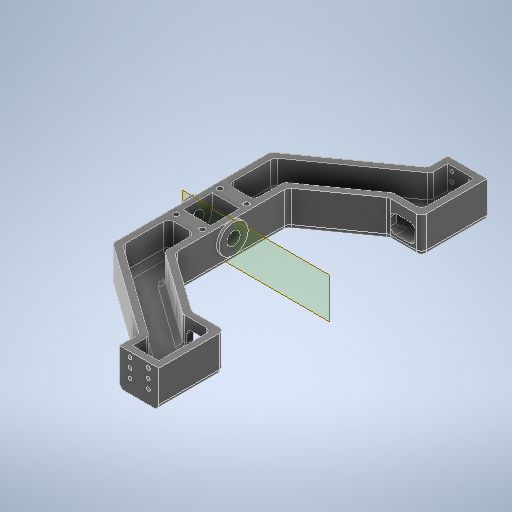
# Autodesk Inventor part: handler_back
Saved by Autodesk Inventor 2025.3 (Build 293356000, 356)
## iProperties
Created: 2026-04-18
Part Number: handler_back
Material: PCTG 20%
Document SubType Name: Modeling
Designer: ksawe
Density: 1.541 g/cm^3
Appearance: Smooth - Black
Author: ksawe
Autodesk Inventor part; units mm, degrees
ref_plane "YZ Plane" through (0, 0, 0) normal (1, 0, 0) x (0, 1, 0)
ref_plane "XZ Plane" through (0, 0, 0) normal (0, 1, 0) x (-1, 0, 0)
sketch "Sketch1" plane through (0, 0, 0) normal (0, 1, 0) x (-1, 0, 0)
  line L0 (-100, 125) -> (-70, 125)
  line L1 (0, 0) -> (-70, 0) construction
  line L2 (-100, 125) -> (-100, 75)
  line L3 (-100, 75) -> (-75, 75)
  line L4 (-70, 125) -> (-70, 110)
  line L5 (-70, 110) -> (0, 60)
  line L6 (0, 60) -> (0, 0)
  line L7 (-75, 75) -> (-30, 42.8571)
  line L8 (-30, 42.8571) -> (-30, 0)
  line L9 (-100, -125) -> (-70, -125)
  line L10 (-100, -125) -> (-100, -75)
  line L11 (-100, -75) -> (-75, -75)
  line L12 (-70, -125) -> (-70, -110)
  line L13 (-70, -110) -> (0, -60)
  line L14 (0, -60) -> (0, 0)
  line L15 (-75, -75) -> (-30, -42.8571)
  line L16 (-30, -42.8571) -> (-30, 0)
  line L17 (-5, 0) -> (-5, 57.4269)
  line L18 (-5, 57.4269) -> (-75, 107.4269)
  line L19 (-75, 107.4269) -> (-75, 120)
  line L20 (-75, 120) -> (-95, 120)
  line L21 (-95, 120) -> (-95, 80)
  line L22 (-95, 80) -> (-73.3977, 80)
  line L23 (-73.3977, 80) -> (-25, 45.4302)
  line L24 (-25, 45.4302) -> (-25, 0)
  line L25 (-25, 0) -> (-25, -45.4302)
  line L26 (-25, -45.4302) -> (-73.3977, -80)
  line L27 (-73.3977, -80) -> (-95, -80)
  line L28 (-95, -80) -> (-95, -120)
  line L29 (-95, -120) -> (-75, -120)
  line L30 (-75, -120) -> (-75, -107.4269)
  line L31 (-75, -107.4269) -> (-5, -57.4269)
  line L32 (-5, -57.4269) -> (-5, 0)
  dimension "d0" = 125
  dimension "d5" = 30
  dimension "d20" = 50
  dimension "d21" = 25
  dimension "d23" = 15
  dimension "d26" = 100
  dimension "d27" = 60
  dimension "d29" = 30
  dimension "d32" = 70
  dimension "d33" = 5
  constraints: 66 end point, 7 symmetric about line, 4 coincident, 4 vertical, 2 horizontal, 2 parallel, 1 horizontal alignment, 15 other
  measures "d0" distance between parallel lines of L1 L0
  measures "d5" distance of L0.start L0.end
  measures "d20" distance of L0.start L2.end
  measures "d21" distance of L2.end L3.end
  measures "d23" distance of L0.end L4.end
  measures "d26" distance between parallel lines of L2 L6
  measures "d27" distance of L5.end L6.end
  measures "d29" distance between parallel lines of L8 L6
  measures "d32" distance of L1.start L1.end
  measures "d33" distance between parallel lines of L6 L17
extrude "Extrusion3" add sketch "Sketch1" against normal blind 6 contours L0 L4 L5 L6 L14 L13 L12 L9 L10 L11 L15 L16 L8 L7 L3 L2 | L32 L31 L30 L29 L28 L27 L26 L25 L24 L23 L22 L21 L20 L19 L18 L17
extrude "Extrusion4" add sketch "Sketch1" along normal blind 22
sketch "Szkic3" plane through (0, 0, 0) normal (0, 1, 0) x (1, 0, 0)
  line L0 (25.5, 11.05) -> (4.5, 11.05)
  line L1 (4.5, 11.05) -> (4.5, -11.05)
  line L2 (4.5, -11.05) -> (25.5, -11.05)
  line L3 (25.5, -11.05) -> (25.5, 11.05)
  line L4 (25.5, 11.05) -> (4.5, -11.05) construction
  line L5 (4.5, 11.05) -> (25.5, -11.05) construction
  line L6 (5, -57.4269) -> (5, 57.4269) projected
  line L7 (5, -22.55) -> (25, -22.55)
  line L8 (25, -45.4302) -> (25, 45.4302) projected
  line L9 (5, 22.55) -> (25, 22.55)
  line L10 (5, 0) -> (25, 0) construction
  point P0 (0, 0)
  point P1 (15, 0)
  point P2 (5, 11.05)
  point P3 (25, 11.05)
  point P4 (25, -11.05)
  point P5 (5, -11.05)
  dimension "d34" = 21
  dimension "d35" = 10
  dimension "d36" = 22.1
  dimension "d37" = 11.5
  constraints: 18 end point, 4 midpoint, 4 point on line, 2 horizontal, 2 parallel, 2 perpendicular, 1 horizontal alignment, 1 other
  measures "d34" distance of L2.end L1.end
  measures "d35" distance from line of L6 point (15, 0)
  measures "d36" distance between parallel lines of L0 L2
  measures "d37" distance between parallel lines of L2 L7
extrude "Wyciągnięcie proste6" add sketch "Szkic3" along normal blind 22 contours L0 L6 L9 L8 | L8 L7 L6 L2
sketch "Szkic4" plane through (30, -6, 42.8571) normal (1, 0, 0) x (0, 0, -1)
  circle A0 centre (42.8571, 16.95) radius 5
  circle A1 centre (42.8571, 16.95) radius 11.05
  line L0 (0, 28) -> (85.7143, 28) projected
  point P0 (42.8571, 6)
  dimension "d40" = 10
  dimension "d41" = 22.1
  constraints: 2 centre point, 2 coincident, 1 tangent, 1 vertical alignment
  measures "d40" diameter of A0
  measures "d41" diameter of A1
extrude "Wyciągnięcie proste7" add sketch "Szkic4" along normal blind 2
extrude "Wyciągnięcie proste8" cut sketch "Szkic4" against normal through all contours A0
ref_plane "Płaszczyzna konstrukcyjna1" through (15, 0, -11.05) normal (1, 0, 0) x (0, 0, -1)
mirror "Odbij1" about plane through (15, 0, -11.05) normal (1, 0, 0) of "Wyciągnięcie proste7"
sketch "Szkic9" plane through (0, 22, 0) normal (0, 1, 0) x (1, 0, 0)
  circle A0 centre (5, -16.8) radius 1.5
  circle A1 centre (5, 16.8) radius 1.5
  circle A2 centre (25, -16.8) radius 1.5
  circle A3 centre (25, 16.8) radius 1.5
  line L0 (25, 11.05) -> (25, -11.05) projected
  line L1 (25, -11.05) -> (5, -11.05) projected
  line L2 (5, -11.05) -> (5, 11.05) projected
  line L3 (5, 11.05) -> (25, 11.05) projected
  line L4 (0, 0) -> (0, -60) projected
  line L5 (5, 0) -> (25, 0)
  line L6 (15, -11.05) -> (15, 11.05)
  dimension "d52" = 3
  dimension "d83" = 5.75
  dimension "d84" = 5
  constraints: 4 centre point, 4 end point, 4 midpoint, 3 other
  measures "d52" diameter of A0
  measures "d83" distance from line of L1 A0.centre
  measures "d84" distance from line of L4 A0.centre
hole "Otwór1" at (5, 22, 16.8) at (25, 22, 16.8) at (25, 22, -16.8) at (5, 22, -16.8) direction (0, -1, 0) diameter 4 depth 7 countersink diameter 4.2 countersink angle 90
sketch "Szkic10" plane through (95, 0, 120) normal (0, 0, -1) x (-1, 0, 0)
  circle A0 centre (3, 18.25) radius 1.5
  line L0 (0, 0) -> (0, 22) projected
  line L1 (0, 22) -> (20, 22) projected
  circle A1 centre (17, 18.25) radius 1.5
  circle A2 centre (3, 11.25) radius 1.5
  circle A3 centre (17, 11.25) radius 1.5
  circle A4 centre (3, 4.25) radius 1.5
  circle A5 centre (17, 4.25) radius 1.5
  line L2 (10, 22) -> (10, 0) construction
  line L3 (20, 0) -> (0, 0) projected
  point P0 (95, 0)
  dimension "d60" = 3
  dimension "d64" = 14
  dimension "d67" = 7
  dimension "d70" = 3.75
  constraints: 6 centre point, 2 end point, 2 midpoint, 1 horizontal, 1 vertical, 11 other
  measures "d60" diameter of A0
  measures "d64" distance of A0.centre A1.centre
  measures "d67" distance of A0.centre A2.centre
  measures "d70" distance from line of L1 A0.centre
extrude "Wyciągnięcie proste11" cut sketch "Szkic10" against normal through all
fillet "Zaokrąglenie1" radius 4 50 edges at (0, -6, 0) (35, -6, -85) (30, -6, 0) (52.5, -6, -58.9286) (52.5, -6, 58.9286) (35, -6, 85) (87.5, -6, -75) (100, -6, -100) (70, -6, -117.5) (87.5, -6, 75) (100, -6, 100) (70, -6, 117.5) (0, 8, 60) (0, 8, -60) (70, 8, -110) (70, 8, 110) (30, 8, -42.8571) (30, 8, 42.8571) (75, 8, 75) (75, 8, -75) (100, 8, -75) (100, 8, 75) (5, 11, -57.4269) (5, 11, 57.4269) (73.3977, 11, 80) (25, 11, 45.4302) (25, 11, -45.4302) (73.3977, 11, -80) (5, 11, -22.55) (25, 11, -22.55) (25, 0, -33.9901) (49.1988, 0, -62.7151) (5, 0, -39.9885) (40, 0, -82.4269) (5, 0, 39.9885) (15, 0, 22.55) (40, 0, 82.4269) (25, 0, 33.9901) (49.1988, 0, 62.7151) (5, 11, 22.55) (25, 11, 22.55) (84.1988, 0, 80) (95, 0, 100) (75, 0, 113.7135) (75, 11, 107.4269) (75, 11, -107.4269) (75, 0, -113.7135) (95, 0, -100) (84.1988, 0, -80) (95, 11, -80)
fillet "Zaokrąglenie2" radius 4 2 edges at (93.8284, 1.1716, 81.1716) (95, 13, 80)
extrude "Extrusion13" cut sketch "Szkic3" along normal up to surface (22 mm away) contours L3 L2 L8 L0 | L6 L2 L1 L0
sketch "Sketch11" plane through (4.5, 0, 11.05) normal (1, 0, 0) x (0, 0, -1)
  circle A0 centre (11.05, 11.05) radius 11.05
  line L0 (22.1, 0) -> (22.1, 22) projected
  line L1 (22.1, 0) -> (0, 0) projected
  line L2 (0, 0) -> (0, 22) projected
  point P0 (11.05, 0)
  point P1 (0, 11.05)
  point P2 (11.05, 0)
  point P3 (22.1, 11.05)
  dimension "d87" = 22.1
  constraints: 2 tangent, 1 centre point
  measures "d87" diameter of A0
extrude "Extrusion14" add sketch "Sketch11" along normal up to surface (21 mm away) contours L0 L1 A0 | A0 L1 L2
sketch "Sketch12" plane through (96, 22, 75) normal (0, 0, -1) x (-1, 0, 0)
  arc A0 (1, -18) -> (5, -22) centre (5, -18) ccw projected
  line L0 (21.3205, -22) -> (5, -22) projected
  line L1 (21.3205, -18) -> (21.3205, 0) projected
  line L2 (19.7181, 0) -> (19.7181, -24) projected
  line L3 (1, -18) -> (1, 0) projected
  line L4 (1, -8) -> (19.7181, -8)
  line L5 (0, 0) -> (19.7181, 0) projected
  point P0 (96, -22)
  point P1 (19.7181, -22)
  dimension "d90" = 8
  constraints: 2 end point, 2 point on line, 1 perpendicular
  measures "d90" distance between parallel lines of L5 L4
extrude "Extrusion15" cut sketch "Sketch12" against normal blind 9 contours L3 L4 L2 L0 A0
fillet "Fillet3" radius 4 3 edges at (76.2819, 14, 77.5) (95, 14, 79.5) (76.2819, 0, 79.5)
ref_plane "Work Plane3" through (25.5, 22, 0) normal (0, 0, -1) x (-1, 0, 0)
mirror "Mirror3" about plane through (25.5, 22, 0) normal (0, 0, -1) of "Fillet3", "Extrusion15", "Wyciągnięcie proste11"
body "Solid2"
